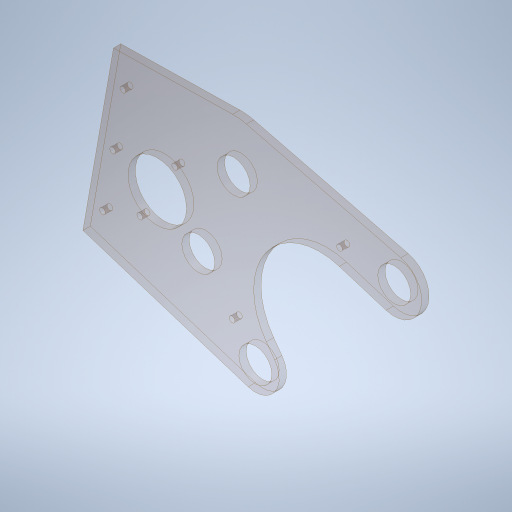
# Autodesk Inventor part: GP7-002
Saved by Autodesk Inventor 2023.4 (Build 274418000, 418)
## iProperties
Created: 2025-02-24
Part Number: GP7-002
Material: Polycarbonate, Smoke
Document SubType Name: Modeling
Designer: dlangdon
Density: 1.2 g/cm^3
Appearance: Polycarbonate - Smoked
Author: dlangdon
Autodesk Inventor part; units mm, degrees
ref_plane "YZ Plane" through (0, 0, 0) normal (1, 0, 0) x (0, 1, 0)
ref_plane "XZ Plane" through (0, 0, 0) normal (0, 1, 0) x (-1, 0, 0)
ref_plane "XY Plane" through (0, 0, 0) normal (0, 0, 1) x (1, 0, 0)
sketch "Sketch1" plane through (0, 0, 0) normal (0, 0, 1) x (1, 0, 0)
  circle A0 centre (64.6578, 64.6578) radius 38.1 construction
  circle A1 centre (-55.6776, -55.6776) radius 25.4 construction
  circle A2 centre (0, 0) radius 53.34 construction
  line L0 (-37.7171, -37.7171) -> (37.7171, 37.7171) construction
  line L1 (64.6578, 64.6578) -> (-55.6776, -55.6776) construction
  line L2 (0, 0) -> (0, 53.34) construction
  line L3 (-213.331, -81.0776) -> (652.061, -81.0776) construction
  circle A3 centre (161.3893, -23.9276) radius 57.15 construction
  circle A4 centre (64.6578, 64.6578) radius 14.2875
  circle A5 centre (-55.6776, -55.6776) radius 14.2875
  circle A6 centre (0, 0) radius 57.15 construction
  circle A7 centre (-55.6776, -55.6776) radius 20.6375 construction
  circle A8 centre (64.6578, 64.6578) radius 23.8125 construction
  circle A9 centre (-74.5156, 76.4795) radius 14.2875
  line L4 (-74.5156, 76.4795) -> (64.6578, 64.6578) construction
  circle A10 centre (64.6578, 64.6578) radius 14.3256 construction
  circle A11 centre (-55.6776, -55.6776) radius 14.3256 construction
  circle A12 centre (-105.1152, 3.2398) radius 14.2875
  line L5 (-55.6776, -55.6776) -> (-105.1152, 3.2398) construction
  circle A13 centre (-105.1152, 3.2398) radius 39.6875 construction
  circle A14 centre (-74.5156, 76.4795) radius 39.6875 construction
  line L6 (16.9977, 54.5637) -> (57.5755, 41.923)
  line L7 (-38.9983, -43.5241) -> (-46.1889, -33.6557)
  arc A15 (16.9977, 54.5637) -> (-46.1889, -33.6557) centre (0, 0) ccw
  line L8 (-178.6215, 120.6011) -> (-153.6074, 116.1905) construction
  line L9 (-153.6074, 116.1905) -> (-180.0714, -33.8943) construction
  line L10 (-180.0714, -33.8943) -> (-205.0855, -29.4836) construction
  line L11 (-205.0855, -29.4836) -> (-178.6215, 120.6011) construction
  line L12 (-209.4704, -54.3516) -> (58.8668, -101.6667) construction
  line L13 (-174.2366, 145.4691) -> (161.1977, 86.323) construction
  line L14 (-174.2366, 145.4691) -> (-209.4704, -54.3516) construction
  circle A16 centre (-140.7036, 31.8148) radius 25.4
  circle A17 centre (-140.7036, 31.8148) radius 5.9531 construction
  line L15 (-79.6045, -27.1626) -> (-72.0044, -36.2201) construction
  circle A18 centre (17.2037, 68.6887) radius 9.525 construction
  line L16 (-166.1144, 118.3958) -> (-192.5784, -31.6889) construction
  line L17 (-170.5251, 93.3817) -> (-188.1678, -6.6748) construction
  circle A19 centre (-140.7036, 31.8148) radius 17.4625 construction
  circle A20 centre (-140.7036, 31.8148) radius 9.525 construction
  circle A21 centre (-74.5156, 76.4795) radius 46.0375 construction
  line L18 (-178.6215, 120.6011) -> (-75.3662, 122.5092)
  line L19 (-63.3695, 121.1474) -> (70.423, 87.7619)
  line L20 (-61.9739, -75.3312) -> (-205.0855, -29.4836)
  line L21 (-178.6215, 120.6011) -> (-205.0855, -29.4836)
  arc A22 (-63.3695, 121.1474) -> (-75.3662, 122.5092) centre (-74.5156, 76.4795) ccw
  arc A23 (57.5755, 41.923) -> (70.423, 87.7619) centre (64.6578, 64.6578) ccw
  arc A24 (-61.9739, -75.3312) -> (-38.9983, -43.5241) centre (-55.6776, -55.6776) ccw
  line L22 (-140.7036, 31.8148) -> (-131.9723, 46.9378) construction
  line L23 (-125.6223, 57.9363) -> (-155.7848, 5.6933) construction
  circle A25 centre (-155.7848, 5.6933) radius 4.7625 construction
  point P0 (-191.8535, 45.5588)
  point P1 (-75.8045, -31.6913)
  point P2 (-179.3464, 43.3534)
  point P3 (-179.3464, 43.3534)
  point P4 (-149.4348, 46.9378)
  point P5 (-158.1661, 31.8148)
  point P6 (-149.4348, 16.6918)
  point P7 (-131.9723, 16.6918)
  point P8 (-123.2411, 31.8148)
  point P9 (-140.7036, 31.8148)
  dimension "d7" = 50.8
  dimension "d18" = 79.375
  dimension "d34" = 34.925
  dimension "d3" = 45
  dimension "d4" = 0
  dimension "d8" = 106.68
  dimension "d9" = 28.575
  dimension "d10" = 76.2
  dimension "d11" = 114.3
  dimension "d12" = 114.3
  dimension "d13" = 6.35
  dimension "d14" = 9.525
  dimension "d15" = 139.6746
  dimension "d16" = 28.6512
  dimension "d17" = 76.9112
  dimension "d19" = 79.375
  dimension "d22" = 25.4
  dimension "d23" = 152.4
  dimension "d26" = 202.9033
  dimension "d27" = 50.8
  dimension "d28" = 11.9062
  dimension "d29" = 50
  dimension "d30" = 171.45
  dimension "d31" = 10
  dimension "d32" = 19.05
  dimension "d33" = 101.6
  dimension "d35" = 19.05
  dimension "d36" = 6.35
  dimension "d37" = 28.575
  dimension "d40" = 360
  dimension "d43" = 20
  dimension "d44" = 9.525
  constraints: 48 end point, 23 centre point, 23 coincident, 19 point on circle, 13 tangent, 9 midpoint, 5 equal radius, 4 collinear, 4 parallel, 4 point on line, 2 horizontal, 1 concentric, 1 perpendicular, 1 vertical, 20 other
  measures "d3" angle of L2 L0
  measures "d4" distance between parallel lines of L0 L1
  measures "d8" diameter of A2
  measures "d9" diameter of A4
  measures "d10" diameter of A0
  measures "d11" diameter of A3
  measures "d12" diameter of A6
  measures "d13" radial gap between concentric circles of A5 A7
  measures "d14" radial gap between concentric circles of A4 A8
  measures "d15" distance of L4.start L4.end
  measures "d16" diameter of A10
  measures "d17" distance of L5.start L5.end
  measures "d19" diameter of A14
  measures "d22" distance of L9.end L10.end
  measures "d23" distance of L10.end L8.start
  measures "d26" distance of L13.start L12.start
  measures "d27" diameter of A16
  measures "d28" diameter of A17
  measures "d29" angle of L3 L5
  measures "d30" distance from line of point (0, 0) L9
  measures "d31" angle of L3 L12
  measures "d32" diameter of A18
  measures "d33" distance of L17.start L17.end
  measures "d35" diameter of A20
  measures "d36" radial gap between concentric circles of A14 A21
  measures "d37" vertical distance of L5.end A16.centre
  measures "d43" angle of L9 L22
  measures "d44" diameter of A25
extrude "Extrusion1" add sketch "Sketch1" along normal blind 6.35
hole "Hole1" at (-75.8045, -31.6913, 0) at (17.2037, 68.6887, 0) at (-170.5251, 93.3817, 0) at (-179.3464, 43.3534, 0) at (-188.1678, -6.6748, 0) at (-131.9723, 46.9378, 0) at (-149.4348, 46.9378, 0) at (-158.1661, 31.8148, 0) at (-149.4348, 16.6918, 0) at (-131.9723, 16.6918, 0) at (-123.2411, 31.8148, 0) at (-125.6223, 57.9363, 0) at (-155.7848, 5.6933, 0) direction (0, 0, 1) diameter 5.1054 end through all clearance for "Flat Head Machine Screw (82)" size "#10" standard "Ansi Unified Screw Threads"
body "Solid1"
